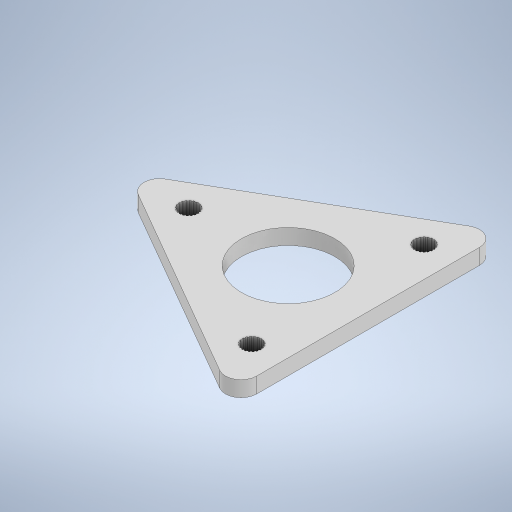
# Autodesk Inventor part: AP-1-01-planetCarrier
Saved by Autodesk Inventor 2024 (Build 280153000, 153)
## iProperties
Created: 2023-07-11
Part Number: AP-1-01-planetCarrier
Material: Generic
Document SubType Name: Modeling
Designer: t205b
Density: 1 g/cm^3
Appearance: Default
Author: t205b
Autodesk Inventor part; units mm, degrees
ref_plane "YZ Plane" through (0, 0, 0) normal (1, 0, 0) x (0, 1, 0)
ref_plane "XZ Plane" through (0, 0, 0) normal (0, 1, 0) x (-1, 0, 0)
ref_plane "XY Plane" through (0, 0, 0) normal (0, 0, 1) x (1, 0, 0)
sketch "Sketch1" plane through (0, 0, 0) normal (0, 1, 0) x (-1, 0, 0)
  line L0 (153.9793, -88.9) -> (0, 0)
  line L1 (0, 0) -> (0, -177.8)
  line L2 (0, -177.8) -> (153.9793, -88.9)
  circle A0 centre (51.3264, -88.9) radius 30
  line L3 (76.9897, -133.35) -> (66.3264, -114.8808) construction
  line L4 (76.9897, -44.45) -> (66.3264, -62.9192) construction
  line L5 (21.3264, -88.9) -> (0, -88.9) construction
  circle A1 centre (115.2355, -88.9) radius 6.1085
  circle A2 centre (19.3719, -144.2469) radius 6.1085
  circle A3 centre (19.3719, -33.5531) radius 6.1085
  line L6 (19.3719, -144.2469) -> (51.3264, -88.9) construction
  line L7 (51.3264, -88.9) -> (115.2355, -88.9) construction
  line L8 (51.3264, -88.9) -> (19.3719, -33.5531) construction
  arc A4 (19.8862, -150.3337) -> (18.8576, -150.3337) centre (19.3719, -150.3604) ccw
  arc A5 (21.7419, -149.8769) -> (20.7637, -150.1947) centre (21.2611, -150.0612) ccw
  arc A6 (23.3657, -148.8689) -> (22.5335, -149.4735) centre (22.9653, -149.1928) ccw
  arc A7 (24.5985, -147.4086) -> (23.9939, -148.2407) centre (24.3178, -147.8403) ccw
  arc A8 (25.3197, -145.6387) -> (25.0019, -146.617) centre (25.1862, -146.1361) ccw
  arc A9 (25.4587, -143.7326) -> (25.4587, -144.7612) centre (25.4854, -144.2469) ccw
  arc A10 (25.0019, -141.8768) -> (25.3197, -142.8551) centre (25.1862, -142.3577) ccw
  arc A11 (23.9939, -140.2531) -> (24.5985, -141.0853) centre (24.3178, -140.6535) ccw
  arc A12 (22.5335, -139.0203) -> (23.3657, -139.6249) centre (22.9653, -139.301) ccw
  arc A13 (20.7637, -138.2991) -> (21.7419, -138.6169) centre (21.2611, -138.4326) ccw
  arc A14 (18.8576, -138.1601) -> (19.8862, -138.1601) centre (19.3719, -138.1334) ccw
  arc A15 (17.0018, -138.6169) -> (17.9801, -138.2991) centre (17.4827, -138.4326) ccw
  arc A16 (15.3781, -139.6249) -> (16.2102, -139.0203) centre (15.7785, -139.301) ccw
  arc A17 (14.1452, -141.0853) -> (14.7499, -140.2531) centre (14.426, -140.6535) ccw
  arc A18 (13.4241, -142.8551) -> (13.7419, -141.8768) centre (13.5576, -142.3577) ccw
  arc A19 (13.2851, -144.7612) -> (13.2851, -143.7326) centre (13.2584, -144.2469) ccw
  arc A20 (13.7419, -146.617) -> (13.4241, -145.6387) centre (13.5576, -146.1361) ccw
  arc A21 (14.7499, -148.2407) -> (14.1452, -147.4086) centre (14.426, -147.8403) ccw
  arc A22 (16.2102, -149.4735) -> (15.3781, -148.8689) centre (15.7785, -149.1928) ccw
  arc A23 (17.9801, -150.1947) -> (17.0018, -149.8769) centre (17.4827, -150.0612) ccw
  arc A24 (121.0824, -87.1314) -> (121.2963, -88.1376) centre (121.2155, -87.6289) ccw
  arc A25 (120.2497, -85.4112) -> (120.764, -86.302) centre (120.53, -85.8432) ccw
  arc A26 (118.9262, -84.0325) -> (119.6906, -84.7208) centre (119.3263, -84.3568) ccw
  arc A27 (117.2414, -83.1302) -> (118.1811, -83.5486) centre (117.7221, -83.315) ccw
  arc A28 (115.3603, -82.7928) -> (116.3833, -82.9003) centre (115.8746, -82.82) ccw
  arc A29 (113.467, -83.0531) -> (114.4731, -82.8393) centre (113.9645, -82.9201) ccw
  arc A30 (111.7467, -83.8858) -> (112.6375, -83.3715) centre (112.1788, -83.6056) ccw
  arc A31 (110.368, -85.2093) -> (111.0563, -84.4449) centre (110.6923, -84.8093) ccw
  arc A32 (109.4658, -86.8941) -> (109.8842, -85.9544) centre (109.6506, -86.4134) ccw
  arc A33 (109.1283, -88.7752) -> (109.2358, -87.7523) centre (109.1555, -88.261) ccw
  arc A34 (113.2297, -94.6698) -> (112.29, -94.2514) centre (112.749, -94.485) ccw
  arc A35 (115.1108, -95.0072) -> (114.0878, -94.8997) centre (114.5965, -94.98) ccw
  arc A36 (117.0041, -94.7469) -> (115.998, -94.9607) centre (116.5066, -94.8799) ccw
  arc A37 (118.7244, -93.9142) -> (117.8336, -94.4285) centre (118.2923, -94.1944) ccw
  arc A38 (120.1031, -92.5907) -> (119.4148, -93.3551) centre (119.7788, -92.9907) ccw
  arc A39 (121.0053, -90.9059) -> (120.5869, -91.8456) centre (120.8205, -91.3866) ccw
  arc A40 (121.3428, -89.0248) -> (121.2353, -90.0477) centre (121.3156, -89.539) ccw
  arc A41 (111.5449, -93.7675) -> (110.7805, -93.0792) centre (111.1448, -93.4432) ccw
  arc A42 (110.2214, -92.3888) -> (109.7071, -91.498) centre (109.9411, -91.9567) ccw
  arc A43 (109.3887, -90.6686) -> (109.1748, -89.6624) centre (109.2556, -90.1711) ccw
  arc A44 (14.9168, -29.3738) -> (15.6812, -28.6856) centre (15.2812, -29.0099) ccw
  arc A45 (13.8434, -30.9551) -> (14.3577, -30.0643) centre (14.0774, -30.4963) ccw
  arc A46 (13.3112, -32.7906) -> (13.525, -31.7845) centre (13.392, -32.282) ccw
  arc A47 (13.3722, -34.7008) -> (13.2647, -33.6778) centre (13.2919, -34.1921) ccw
  arc A48 (14.0205, -36.4987) -> (13.6021, -35.559) centre (13.7869, -36.0397) ccw
  arc A49 (15.1926, -38.0082) -> (14.5044, -37.2438) centre (14.8287, -37.6438) ccw
  arc A50 (16.7739, -39.0816) -> (15.8831, -38.5673) centre (16.3151, -38.8475) ccw
  arc A51 (18.6094, -39.6138) -> (17.6033, -39.4) centre (18.1008, -39.533) ccw
  arc A52 (20.5196, -39.5528) -> (19.4966, -39.6603) centre (20.0109, -39.6331) ccw
  arc A53 (22.3175, -38.9045) -> (21.3778, -39.3229) centre (21.8585, -39.138) ccw
  arc A54 (25.3716, -32.4054) -> (25.4791, -33.4283) centre (25.4519, -32.9141) ccw
  arc A55 (24.7233, -30.6075) -> (25.1416, -31.5472) centre (24.9568, -31.0665) ccw
  arc A56 (23.5511, -29.098) -> (24.2394, -29.8624) centre (23.9151, -29.4624) ccw
  arc A57 (21.9699, -28.0246) -> (22.8607, -28.5389) centre (22.4286, -28.2586) ccw
  arc A58 (20.1343, -27.4924) -> (21.1405, -27.7062) centre (20.643, -27.5732) ccw
  arc A59 (18.2241, -27.5534) -> (19.2471, -27.4459) centre (18.7328, -27.4731) ccw
  arc A60 (16.4263, -28.2017) -> (17.366, -27.7833) centre (16.8853, -27.9681) ccw
  arc A61 (25.4326, -34.3155) -> (25.2188, -35.3217) centre (25.3518, -34.8242) ccw
  arc A62 (24.9004, -36.1511) -> (24.3861, -37.0419) centre (24.6663, -36.6098) ccw
  arc A63 (23.827, -37.7323) -> (23.0625, -38.4206) centre (23.4626, -38.0963) ccw
  point P0 (21.7419, -149.8769)
  point P1 (23.3657, -148.8689)
  point P2 (22.5335, -149.4735)
  point P3 (24.5985, -147.4086)
  point P4 (25.0019, -141.8768)
  point P5 (25.3197, -142.8551)
  point P6 (23.9939, -140.2531)
  point P7 (22.5335, -139.0203)
  point P8 (23.3657, -139.6249)
  point P9 (20.7637, -138.2991)
  point P10 (21.7419, -138.6169)
  point P11 (19.8862, -138.1601)
  point P12 (17.9801, -138.2991)
  point P13 (15.3781, -139.6249)
  point P14 (16.2102, -139.0203)
  point P15 (14.1452, -141.0853)
  point P16 (14.7499, -140.2531)
  point P17 (13.2851, -144.7612)
  point P18 (13.7419, -146.617)
  point P19 (13.4241, -145.6387)
  point P20 (14.7499, -148.2407)
  point P21 (14.1452, -147.4086)
  point P22 (16.2102, -149.4735)
  point P23 (15.3781, -148.8689)
  point P24 (17.0018, -149.8769)
  point P25 (15.6812, -28.6856)
  point P26 (13.8434, -30.9551)
  point P27 (14.3577, -30.0643)
  point P28 (13.3112, -32.7906)
  point P29 (13.525, -31.7845)
  point P30 (14.0205, -36.4987)
  point P31 (15.1926, -38.0082)
  point P32 (14.5044, -37.2438)
  point P33 (16.7739, -39.0816)
  point P34 (15.8831, -38.5673)
  point P35 (18.6094, -39.6138)
  point P36 (17.6033, -39.4)
  point P37 (20.5196, -39.5528)
  point P38 (19.4966, -39.6603)
  point P39 (22.3175, -38.9045)
  point P40 (21.3778, -39.3229)
  point P41 (25.3716, -32.4054)
  point P42 (25.4791, -33.4283)
  point P43 (24.7233, -30.6075)
  point P44 (25.1416, -31.5472)
  point P45 (23.5511, -29.098)
  point P46 (24.2394, -29.8624)
  point P47 (21.9699, -28.0246)
  point P48 (22.8607, -28.5389)
  point P49 (20.1343, -27.4924)
  point P50 (21.1405, -27.7062)
  point P51 (18.2241, -27.5534)
  point P52 (16.4263, -28.2017)
  point P53 (17.366, -27.7833)
  point P54 (25.2188, -35.3217)
  point P55 (24.9004, -36.1511)
  point P56 (24.3861, -37.0419)
  point P57 (23.827, -37.7323)
  point P58 (23.0625, -38.4206)
  point P59 (121.0824, -87.1314)
  point P60 (120.764, -86.302)
  point P61 (118.1811, -83.5486)
  point P62 (115.3603, -82.7928)
  point P63 (116.3833, -82.9003)
  point P64 (111.7467, -83.8858)
  point P65 (112.6375, -83.3715)
  point P66 (109.8842, -85.9544)
  point P67 (109.2358, -87.7523)
  point P68 (121.3428, -89.0248)
  point P69 (110.2214, -92.3888)
  point P70 (109.7071, -91.498)
  point P71 (109.3887, -90.6686)
  point P72 (109.1748, -89.6624)
  point P73 (113.2297, -94.6698)
  point P74 (112.29, -94.2514)
  point P75 (115.1108, -95.0072)
  point P76 (117.0041, -94.7469)
  point P77 (117.8336, -94.4285)
  point P78 (119.4148, -93.3551)
  dimension "d4" = 12.217
  dimension "d0" = 177.8
  dimension "d1" = 60
  dimension "d2" = 102.6529
  dimension "d3" = 63.9091
  dimension "d5" = 120
  dimension "d6" = 120
  dimension "d11" = 0.515
  dimension "d12" = 6.1135
  dimension "d15" = 360
  dimension "d19" = 360
  constraints: 123 point on circle, 61 centre point, 18 end point, 6 equal length, 3 line through centre, 3 midpoint, 2 perpendicular, 1 coincident, 1 horizontal, 1 vertical, 1 vertical alignment, 330 other
  measures "d0" distance of L0.end L1.end
  measures "d1" diameter of A0
  measures "d2" distance of L1.end L6.end
  measures "d3" distance of L6.start L6.end
  measures "d5" angle of L6 L7
  measures "d6" angle of L8 L7
  measures "d11" radius of A4
  measures "d12" distance of A4.centre L6.start
extrude "Extrusion1" add sketch "Sketch1" along normal blind 10 contours L2 L1 L0 | A24 A1 | A1 A40 | A25 A1 | A1 A39 | A26 A1 | A1 A38 | A27 A1 | A1 A37 | A28 A1 | A1 A36 | A29 A1 | A1 A35 | A30 A1 | A1 A34 | A31 A1 | A1 A41 | A32 A1 | A1 A42 | A33 A1 | A1 A43 | A2 A9 | A10 A2 | A2 A8 | A11 A2 | A2 A7 | A12 A2 | A2 A6 | A13 A2 | A2 A5 | A14 A2 | A2 A4 | A15 A2 | A2 A23 | A16 A2 | A2 A22 | A17 A2 | A2 A21 | A18 A2 | A2 A20 | A19 A2 | A54 A3 | A3 A61 | A55 A3 | A3 A62 | A56 A3 | A3 A63 | A57 A3 | A3 A53 | A58 A3 | A3 A52 | A59 A3 | A3 A51 | A60 A3 | A3 A50 | A44 A3 | A3 A49 | A45 A3 | A3 A48 | A46 A3 | A3 A47
fillet "Fillet1" radius 10 3 edges at (0, 5, -177.8) (0, 5, 0) (-153.9793, 5, -88.9)
body "Solid1"
